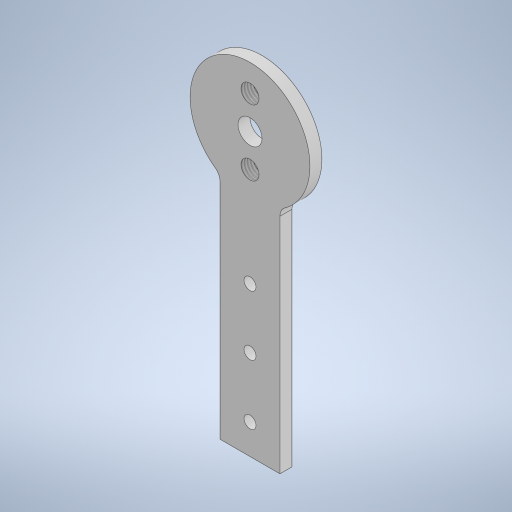
# Autodesk Inventor part: cutter_board
Saved by Autodesk Inventor 2024 (Build 280153000, 153)
## iProperties
Created: 2025-03-05
Part Number: cutter_board
Material: 一般
Document SubType Name: Modeling
Designer: 1412z
Density: 1 g/cm^3
Appearance: 既定
Author: 1412z
Autodesk Inventor part; units mm, degrees
ref_plane "YZ Plane" through (0, 0, 0) normal (1, 0, 0) x (0, 1, 0)
ref_plane "XZ Plane" through (0, 0, 0) normal (0, 1, 0) x (-1, 0, 0)
ref_plane "XY Plane" through (0, 0, 0) normal (0, 0, 1) x (1, 0, 0)
sketch "スケッチ1" plane through (0, 0, 0) normal (0, 0, 1) x (1, 0, 0)
  circle A0 centre (0, 0) radius 10
  circle A1 centre (0, 0) radius 2
  line L0 (0, -2) -> (0, -47)
  line L1 (10, 0) -> (10, -47)
  line L2 (10, -47) -> (-10, -47)
  line L3 (-10, -47) -> (-10, 0)
  circle A2 centre (0, -32) radius 1
  circle A3 centre (0, -42) radius 1
  circle A4 centre (0, -22) radius 1
  dimension "d1" = 4
  dimension "d0" = 20
  dimension "d2" = 45
  dimension "d9" = 2
  dimension "d10" = 2
  dimension "d11" = 2
  constraints: 8 end point, 4 centre point, 3 point on line, 2 coincident, 2 point on circle, 2 tangent, 2 vertical, 1 perpendicular, 1 vertical alignment, 2 other
  measures "d0" diameter of A0
  measures "d2" distance of L0.start L0.end
  measures "d9" diameter of A2
  measures "d10" diameter of A3
  measures "d11" diameter of A4
extrude "押し出し1" add sketch "スケッチ1" along normal blind 2
sketch "スケッチ2" plane through (0, 0, 2) normal (0, 0, 1) x (1, 0, 0)
  circle A0 centre (0, -32) radius 1
  circle A1 centre (0, -22) radius 1
  circle A2 centre (0, -42) radius 1
  point P0 (0, 0)
  dimension "d12" = 2
  dimension "d13" = 2
  dimension "d14" = 2
  constraints: 3 centre point
  measures "d12" diameter of A0
  measures "d13" diameter of A1
  measures "d14" diameter of A2
extrude "押し出し2" cut sketch "スケッチ2" against normal blind 10
sketch "スケッチ3" plane through (0, 0, 0) normal (0, 0, -1) x (-1, 0, 0)
  line L0 (10, -47) -> (-10, -47) projected
  line L1 (10, -47) -> (5, -47)
  circle A0 centre (0, 0) radius 10
  line L2 (5, -47) -> (5, -8.6603)
  line L3 (10, 0) -> (10, -47) projected
  line L4 (10, -47) -> (10, 0)
  line L5 (-10, -47) -> (-10, 0) projected
  line L6 (-10, 0) -> (-10, -47)
  line L7 (-10, -47) -> (-5, -47)
  line L8 (-5, -47) -> (-5, -8.6603)
  dimension "d17" = 5
  dimension "d18" = 5
  constraints: 12 end point, 3 point on circle, 2 collinear, 2 point on line, 1 centre point, 1 coincident, 1 perpendicular, 1 tangent
  measures "d17" distance of L0.start L1.end
  measures "d18" distance of L0.end L7.end
extrude "押し出し3" cut sketch "スケッチ3" against normal blind 10 contours L0 L2 A0 L3 | L0 L5 A0 L8
sketch "スケッチ4" plane through (0, 0, 0) normal (0, 0, -1) x (-1, 0, 0)
  circle A0 centre (0, 0) radius 5.5
  circle A1 centre (0, -5.5) radius 1.5
  circle A2 centre (0, 5.5) radius 1.5
  dimension "d21" = 11
  dimension "d22" = 3
  dimension "d23" = 3
  constraints: 3 centre point, 2 point on circle, 1 coincident
  measures "d21" diameter of A0
  measures "d22" diameter of A1
  measures "d23" diameter of A2
extrude "押し出し4" cut sketch "スケッチ4" against normal blind 10 contours A2 A0 | A0 A2 | A1 A0 | A0 A1
thread "ねじ1" size "M3x0.5" class "6H" standard "ANSI Metric M Profile" full length
thread "ねじ2" size "M3x0.5" class "6H" standard "ANSI Metric M Profile" full length
fillet "フィレット1" radius 2 2 edges at (5, -8.6603, 1) (-5, -8.6603, 1)
